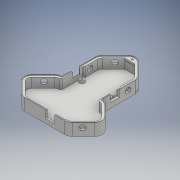
# Autodesk Inventor part: DynamicClampBottomMegaCompact
Saved by Autodesk Inventor 2017 (Build 210142000, 142)
## iProperties
Created: 2017-11-01
Part Number: DynamicClampBottomMegaCompact
Material: Generic
Document SubType Name: Modeling
Designer: andrew
Density: 1 g/cm^3
Appearance: Default
Author: andrew
Autodesk Inventor part; units mm, degrees
ref_plane "YZ Plane" through (0, 0, 0) normal (1, 0, 0) x (0, 1, 0)
ref_plane "XZ Plane" through (0, 0, 0) normal (0, 1, 0) x (-1, 0, 0)
ref_plane "XY Plane" through (0, 0, 0) normal (0, 0, 1) x (1, 0, 0)
sketch "Sketch1" plane through (0, 0, 0) normal (0, 0, 1) x (1, 0, 0)
  line L0 (64.8995, 131.8825) -> (42.1924, 154.5896)
  arc A0 (42.1924, 154.5896) -> (23.8076, 154.5896) centre (33, 145.3972) ccw
  line L1 (23.8076, 154.5896) -> (1.1005, 131.8825)
  line L2 (-3, -3) -> (69, -3) construction
  arc A1 (4.3647, 133.7325) -> (4.35, 133.7177) centre (12.85, 125.2472) ccw
  line L3 (69, 102) -> (69, 121.983)
  line L4 (-3, -3) -> (69, -3)
  arc A2 (1.1005, 131.8825) -> (-3, 121.983) centre (11, 121.983) ccw
  arc A3 (69, 121.983) -> (64.8995, 131.8825) centre (55, 121.983) ccw
  line L5 (-12.1924, 0.8076) -> (-32.3424, 20.9576)
  line L6 (-25.6012, -1.7073) -> (-34.8573, 7.5488) construction
  arc A4 (-32.3424, 39.3424) -> (-32.3424, 20.9576) centre (-23.15, 30.15) ccw
  line L7 (-32.3424, 39.3424) -> (-12.1924, 59.4924)
  arc A5 (-3, 63.3) -> (-12.1924, 59.4924) centre (-3, 50.3) ccw
  arc A6 (-12.1924, 0.8076) -> (-3, -3) centre (-3, 10) ccw
  line L8 (78.1924, 59.4924) -> (98.3424, 39.3424)
  arc A7 (98.3424, 20.9576) -> (98.3424, 39.3424) centre (89.15, 30.15) ccw
  line L9 (98.3424, 20.9576) -> (78.1924, 0.8076)
  arc A8 (69, -3) -> (78.1924, 0.8076) centre (69, 10) ccw
  arc A9 (78.1924, 59.4924) -> (69, 63.3) centre (69, 50.3) ccw
  line L10 (69, 102) -> (69, 63.3)
  line L11 (-3, 121.983) -> (-3, 63.3)
  point P0 (-37.2921, 30.15)
  point P1 (103.2921, 30.15)
  point P2 (73.1421, 60.3)
  constraints: 24 end point, 20 point on circle, 10 centre point, 3 tangent, 3 vertical, 1 collinear, 1 equal radius
extrude "Extrusion1" add sketch "Sketch1" along normal blind 3
sketch "Sketch2" plane through (0, 0, 3) normal (0, 0, 1) x (1, 0, 0)
  line L0 (65.9995, 1.253) -> (32.9995, 1.253) construction
  line L1 (32.9995, 1.253) -> (64.747, 1.253) construction
  line L2 (64.7475, 0) -> (64.7475, 1.253) construction
  line L3 (64.7475, 1.253) -> (60.9425, 1.253) construction
  line L4 (3.8431, 128.2611) -> (24.1624, 148.5804)
  line L5 (23.8076, 154.5896) -> (1.1005, 131.8825)
  line L6 (41.8376, 148.5804) -> (24.1624, 148.5804)
  line L7 (41.8376, 148.5804) -> (62.1569, 128.2611)
  line L8 (64.8995, 131.8825) -> (42.1924, 154.5896)
  arc A0 (42.1924, 154.5896) -> (23.8076, 154.5896) centre (33, 145.3972) ccw
  line L9 (-3, -3) -> (69, -3) construction
  line L10 (-3, 99) -> (0, 99) construction
  arc A1 (1.252, 128.3272) -> (1.2515, 128.3253) centre (12.85, 125.2472) ccw
  arc A2 (0.85, 125.268) -> (0.85, 125.2472) centre (12.85, 125.2472) ccw
  arc A3 (4.3647, 133.7325) -> (4.35, 133.7177) centre (12.85, 125.2472) ccw
  line L11 (1.5, 100.5) -> (1.5, 122.6043)
  line L12 (69, 102) -> (69, 121.983)
  line L13 (64.5, 122.6043) -> (64.5, 100.5)
  line L14 (64.5, 99) -> (69, 99) construction
  line L15 (-3, -3) -> (69, -3)
  line L16 (66, 99) -> (66, 99)
  arc A4 (3.8431, 128.2611) -> (1.5, 122.6043) centre (9.5, 122.6043) ccw
  arc A5 (64.5, 122.6043) -> (62.1569, 128.2611) centre (56.5, 122.6043) ccw
  arc A6 (1.1005, 131.8825) -> (-3, 121.983) centre (11, 121.983) ccw
  arc A7 (69, 121.983) -> (64.8995, 131.8825) centre (55, 121.983) ccw
  arc A8 (0.75, 99.201) -> (1.5, 100.5) centre (0, 100.5) ccw
  arc A9 (0.75, 99.201) -> (0, 97.9019) centre (1.5, 97.9019) ccw
  arc A10 (64.5, 100.5) -> (65.25, 99.201) centre (66, 100.5) ccw
  arc A11 (66, 97.9019) -> (65.25, 99.201) centre (64.5, 97.9019) ccw
  line L17 (65.9995, 1.253) -> (32.9995, 1.253) construction
  line L18 (32.9995, 1.253) -> (64.747, 1.253) construction
  line L19 (64.7475, 0) -> (64.7475, 1.253) construction
  line L20 (64.7475, 1.253) -> (60.9425, 1.253) construction
  line L21 (3.8431, 128.2611) -> (24.1624, 148.5804)
  line L22 (23.8076, 154.5896) -> (1.1005, 131.8825)
  line L23 (41.8376, 148.5804) -> (24.1624, 148.5804)
  line L24 (41.8376, 148.5804) -> (62.1569, 128.2611)
  line L25 (64.8995, 131.8825) -> (42.1924, 154.5896)
  arc A12 (42.1924, 154.5896) -> (23.8076, 154.5896) centre (33, 145.3972) ccw
  line L26 (-3, -3) -> (69, -3) construction
  line L27 (-3, 99) -> (0, 99) construction
  arc A13 (1.252, 128.3272) -> (1.2515, 128.3253) centre (12.85, 125.2472) ccw
  arc A14 (0.85, 125.268) -> (0.85, 125.2472) centre (12.85, 125.2472) ccw
  arc A15 (4.3647, 133.7325) -> (4.35, 133.7177) centre (12.85, 125.2472) ccw
  line L28 (1.5, 100.5) -> (1.5, 122.6043)
  line L29 (69, 102) -> (69, 121.983)
  line L30 (64.5, 122.6043) -> (64.5, 100.5)
  line L31 (64.5, 99) -> (69, 99) construction
  line L32 (-3, -3) -> (69, -3)
  line L33 (66, 99) -> (66, 99)
  arc A16 (3.8431, 128.2611) -> (1.5, 122.6043) centre (9.5, 122.6043) ccw
  arc A17 (64.5, 122.6043) -> (62.1569, 128.2611) centre (56.5, 122.6043) ccw
  arc A18 (1.1005, 131.8825) -> (-3, 121.983) centre (11, 121.983) ccw
  arc A19 (69, 121.983) -> (64.8995, 131.8825) centre (55, 121.983) ccw
  arc A20 (0.75, 99.201) -> (1.5, 100.5) centre (0, 100.5) ccw
  arc A21 (0.75, 99.201) -> (0, 97.9019) centre (1.5, 97.9019) ccw
  arc A22 (64.5, 100.5) -> (65.25, 99.201) centre (66, 100.5) ccw
  arc A23 (66, 97.9019) -> (65.25, 99.201) centre (64.5, 97.9019) ccw
  line L34 (-19.0039, 14.1461) -> (-22.5076, 17.6498) construction
  arc A24 (-9.0104, 3.9896) -> (-3, 1.5) centre (-3, 10) ccw
  line L35 (-34.8573, 7.5488) -> (-12.4066, 29.9994) construction
  line L36 (-9.0104, 3.9896) -> (-29.1604, 24.1396)
  line L37 (-12.1924, 0.8076) -> (-32.3424, 20.9576)
  line L38 (-25.6012, -1.7073) -> (-34.8573, 7.5488) construction
  line L39 (-23.6319, 18.7741) -> (-14.3759, 9.5181) construction
  arc A25 (-12.1924, 0.8076) -> (-3, -3) centre (-3, 10) ccw
  arc A26 (-29.1604, 36.1604) -> (-29.1604, 24.1396) centre (-23.15, 30.15) ccw
  line L40 (-26.3333, 21.3124) -> (-26.3333, 38.9876) construction
  arc A27 (-32.3424, 39.3424) -> (-32.3424, 20.9576) centre (-23.15, 30.15) ccw
  line L41 (-19.0854, 14.0646) -> (-26.3333, 21.3124) construction
  line L42 (-29.1604, 36.1604) -> (-9.0104, 56.3104)
  line L43 (-32.3424, 39.3424) -> (-12.1924, 59.4924)
  arc A28 (-3, 58.8) -> (-9.0104, 56.3104) centre (-3, 50.3) ccw
  line L44 (-8.387, 60.3) -> (4.703, 60.3) construction
  arc A29 (-3, 63.3) -> (-12.1924, 59.4924) centre (-3, 50.3) ccw
  line L45 (88.5076, 42.6502) -> (77.2823, 31.4249) construction
  line L46 (85.0039, 46.1539) -> (88.5076, 42.6502) construction
  arc A30 (75.0104, 56.3104) -> (69, 58.8) centre (69, 50.3) ccw
  line L47 (100.8573, 52.7512) -> (78.4066, 30.3006) construction
  line L48 (78.1924, 59.4924) -> (98.3424, 39.3424)
  line L49 (91.6012, 62.0073) -> (100.8573, 52.7512) construction
  arc A31 (78.1924, 59.4924) -> (69, 63.3) centre (69, 50.3) ccw
  arc A32 (95.1604, 24.1396) -> (95.1604, 36.1604) centre (89.15, 30.15) ccw
  line L50 (92.3333, 38.9876) -> (92.3333, 21.3124) construction
  arc A33 (98.3424, 20.9576) -> (98.3424, 39.3424) centre (89.15, 30.15) ccw
  line L51 (85.0854, 46.2354) -> (92.3333, 38.9876) construction
  line L52 (95.1604, 24.1396) -> (75.0104, 3.9896)
  line L53 (98.3424, 20.9576) -> (78.1924, 0.8076)
  arc A34 (69, 1.5) -> (75.0104, 3.9896) centre (69, 10) ccw
  line L54 (74.387, 0) -> (61.297, 0) construction
  arc A35 (69, -3) -> (78.1924, 0.8076) centre (69, 10) ccw
  line L55 (69, 1.5) -> (66, 0)
  line L56 (69, 58.8) -> (66, 58.8)
  line L57 (-3, 58.8) -> (0, 58.8)
  line L58 (-3, -3) -> (-3, -1.8579)
  line L59 (75.0104, 56.3104) -> (95.1604, 36.1604)
  line L60 (-3, 1.5) -> (0, 0)
  line L61 (0, 0) -> (66, 0)
  line L62 (118.9961, 116.6519) -> (118.9961, 98.6519)
  line L63 (118.9961, 116.6519) -> (136.9961, 116.6519) construction
  line L64 (0, 97.9019) -> (0, 58.8)
  line L65 (-3, 63.3) -> (-3, 121.983)
  line L66 (69, 102) -> (69, 63.3)
  line L67 (66, 97.9019) -> (66, 58.8)
  point P0 (-7.1421, 0)
  point P1 (-37.2921, 30.15)
  point P2 (73.1421, 60.3)
  point P3 (103.2921, 30.15)
  dimension "d28" = 8
  dimension "d126" = 8
  dimension "d186" = 18
  dimension "d187" = 90
  constraints: 136 end point, 76 point on circle, 36 centre point, 27 tangent, 11 point on line, 9 vertical, 8 equal radius, 5 horizontal, 3 collinear, 3 midpoint, 2 parallel, 2 perpendicular, 6 other
  measures "d28" radius of A4
  measures "d126" radius of A16
  measures "d186" distance of L62.start L62.end
  measures "d187" angle of L62 L63
extrude "Extrusion2" add sketch "Sketch2" along normal blind 17.3 contours A4 L11 A1 L4 | A0 L8 A7 L12 L66 A31 L48 A33 L53 A35 L15 A25 L37 A27 L43 A29 L65 A6 L5 picked at (9.0553, 134.1739)
sketch "Sketch3" plane through (0, 0, 20.3) normal (0, 0, 1) x (1, 0, 0)
  line L0 (66, 58.8) -> (69, 58.8) projected
  arc A0 (75.0104, 56.3104) -> (69, 58.8) centre (69, 50.3) ccw projected
  line L1 (75.0104, 56.3104) -> (95.1604, 36.1604) projected
  arc A1 (95.1604, 24.1396) -> (95.1604, 36.1604) centre (89.15, 30.15) ccw projected
  line L2 (95.1604, 24.1396) -> (75.0104, 3.9896) projected
  arc A2 (69, 1.5) -> (75.0104, 3.9896) centre (69, 10) ccw projected
  line L3 (69, 1.5) -> (66, 0) projected
  line L4 (66, 0) -> (0, 0) projected
  line L5 (0, 0) -> (-3, 1.5) projected
  arc A3 (-9.0104, 3.9896) -> (-3, 1.5) centre (-3, 10) ccw projected
  line L6 (-9.0104, 3.9896) -> (-29.1604, 24.1396) projected
  arc A4 (-29.1604, 36.1604) -> (-29.1604, 24.1396) centre (-23.15, 30.15) ccw projected
  line L7 (-29.1604, 36.1604) -> (-9.0104, 56.3104) projected
  arc A5 (-3, 58.8) -> (-9.0104, 56.3104) centre (-3, 50.3) ccw projected
  line L8 (-3, 58.8) -> (0, 58.8) projected
  arc A6 (-3, 63.3) -> (-12.1924, 59.4924) centre (-3, 50.3) ccw projected
  line L9 (-12.1924, 59.4924) -> (-32.3424, 39.3424) projected
  arc A7 (-32.3424, 39.3424) -> (-32.3424, 20.9576) centre (-23.15, 30.15) ccw projected
  line L10 (-32.3424, 20.9576) -> (-12.1924, 0.8076) projected
  arc A8 (-12.1924, 0.8076) -> (-3, -3) centre (-3, 10) ccw projected
  line L11 (-3, -3) -> (69, -3) projected
  arc A9 (69, -3) -> (78.1924, 0.8076) centre (69, 10) ccw projected
  line L12 (78.1924, 0.8076) -> (98.3424, 20.9576) projected
  arc A10 (98.3424, 20.9576) -> (98.3424, 39.3424) centre (89.15, 30.15) ccw projected
  line L13 (98.3424, 39.3424) -> (78.1924, 59.4924) projected
  arc A11 (78.1924, 59.4924) -> (69, 63.3) centre (69, 50.3) ccw projected
  line L14 (0, 58.8) -> (0, 97.9019) projected
  arc A12 (0.75, 99.201) -> (0, 97.9019) centre (1.5, 97.9019) ccw projected
  arc A13 (0.75, 99.201) -> (1.5, 100.5) centre (0, 100.5) ccw projected
  line L15 (1.5, 100.5) -> (1.5, 122.6043) projected
  arc A14 (3.8431, 128.2611) -> (1.5, 122.6043) centre (9.5, 122.6043) ccw projected
  line L16 (3.8431, 128.2611) -> (24.1624, 148.5804) projected
  line L17 (24.1624, 148.5804) -> (41.8376, 148.5804) projected
  line L18 (41.8376, 148.5804) -> (62.1569, 128.2611) projected
  arc A15 (64.5, 122.6043) -> (62.1569, 128.2611) centre (56.5, 122.6043) ccw projected
  line L19 (64.5, 122.6043) -> (64.5, 100.5) projected
  arc A16 (64.5, 100.5) -> (65.25, 99.201) centre (66, 100.5) ccw projected
  arc A17 (66, 97.9019) -> (65.25, 99.201) centre (64.5, 97.9019) ccw projected
  line L20 (66, 97.9019) -> (66, 58.8) projected
  arc A18 (42.1924, 154.5896) -> (23.8076, 154.5896) centre (33, 145.3972) ccw projected
  line L21 (23.8076, 154.5896) -> (1.1005, 131.8825) projected
  arc A19 (1.1005, 131.8825) -> (-3, 121.983) centre (11, 121.983) ccw projected
  line L22 (-3, 121.983) -> (-3, 63.3) projected
  line L23 (69, 63.3) -> (69, 121.983) projected
  arc A20 (69, 121.983) -> (64.8995, 131.8825) centre (55, 121.983) ccw projected
  line L24 (64.8995, 131.8825) -> (42.1924, 154.5896) projected
  arc A21 (-2, 62.2583) -> (-11.4853, 58.7853) centre (-3, 50.3) ccw
  line L25 (-11.4853, 58.7853) -> (-31.6353, 38.6353)
  arc A22 (-31.6353, 38.6353) -> (-31.6353, 21.6647) centre (-23.15, 30.15) ccw
  line L26 (-31.6353, 21.6647) -> (-11.4853, 1.5147)
  arc A23 (-11.4853, 1.5147) -> (-3, -2) centre (-3, 10) ccw
  line L27 (-3, -2) -> (69, -2)
  arc A24 (69, -2) -> (77.4853, 1.5147) centre (69, 10) ccw
  line L28 (77.4853, 1.5147) -> (97.6353, 21.6647)
  arc A25 (97.6353, 21.6647) -> (97.6353, 38.6353) centre (89.15, 30.15) ccw
  line L29 (97.6353, 38.6353) -> (77.4853, 58.7853)
  arc A26 (77.4853, 58.7853) -> (68, 62.2583) centre (69, 50.3) ccw
  line L30 (68, 62.2583) -> (68, 121.983)
  arc A27 (68, 121.983) -> (64.1924, 131.1754) centre (55, 121.983) ccw
  line L31 (64.1924, 131.1754) -> (41.4853, 153.8825)
  arc A28 (41.4853, 153.8825) -> (24.5147, 153.8825) centre (33, 145.3972) ccw
  line L32 (24.5147, 153.8825) -> (1.8076, 131.1754)
  arc A29 (1.8076, 131.1754) -> (-2, 121.983) centre (11, 121.983) ccw
  line L33 (-2, 121.983) -> (-2, 62.2583)
  dimension "d188" = 1
  constraints: 18 end point, 18 point on circle, 9 centre point, 17 other
  measures "d188" distance between parallel lines of L22 L33
extrude "Extrusion3" add sketch "Sketch3" along normal blind 1 contours L22 A19 L21 A18 L24 A20 L23 A11 L13 A10 L12 A9 L11 A8 L10 A7 L9 A6
sketch "Sketch4" plane through (0, 0, 3) normal (0, 0, 1) x (1, 0, 0)
  line L0 (0, 0) -> (66, 0) construction
  line L1 (66, 0) -> (66, 117) construction
  line L2 (0, 115.9019) -> (0, 0) construction
  line L3 (66, 115.9019) -> (66, 60.5) construction
  line L4 (65.9995, 1.253) -> (32.9995, 1.253) construction
  line L5 (32.9995, 1.253) -> (64.747, 1.253) construction
  line L6 (64.747, 1.253) -> (64.747, 48.238) construction
  line L7 (64.7475, 0) -> (64.7475, 1.253) construction
  line L8 (64.7475, 1.253) -> (60.9425, 1.253) construction
  line L9 (60.9425, 1.253) -> (60.9425, 5.058) construction
  line L10 (60.9425, 5.058) -> (64.7475, 5.058) construction
  line L11 (64.7475, 5.058) -> (64.7475, 1.253) construction
  circle A0 centre (60.9425, 5.058) radius 1.6
  line L12 (64.747, 95.223) -> (64.747, 48.238) construction
  line L13 (60.9425, 91.418) -> (64.7475, 91.418) construction
  circle A1 centre (60.9425, 91.418) radius 1.6
  line L14 (64.7475, 91.418) -> (64.7475, 95.223) construction
  line L15 (64.7475, 95.223) -> (60.9425, 95.223) construction
  line L16 (60.9425, 95.223) -> (60.9425, 91.418) construction
  line L17 (64.7475, 96.476) -> (64.7475, 95.223) construction
  line L18 (65.9995, 95.223) -> (32.9995, 95.223) construction
  line L19 (32.9995, 95.223) -> (64.747, 95.223) construction
  line L20 (32.9995, 95.223) -> (1.252, 95.223) construction
  line L21 (-0.0005, 95.223) -> (32.9995, 95.223) construction
  line L22 (1.2515, 91.418) -> (1.2515, 95.223) construction
  line L23 (5.0565, 91.418) -> (1.2515, 91.418) construction
  line L24 (5.0565, 95.223) -> (5.0565, 91.418) construction
  circle A2 centre (5.0565, 91.418) radius 1.6
  line L25 (1.252, 95.223) -> (1.252, 48.238) construction
  line L26 (-0.0005, 1.253) -> (32.9995, 1.253) construction
  line L27 (32.9995, 1.253) -> (1.252, 1.253) construction
  line L28 (1.252, 1.253) -> (1.252, 48.238) construction
  line L29 (5.0565, 5.058) -> (1.2515, 5.058) construction
  circle A3 centre (5.0565, 5.058) radius 1.6
  line L30 (5.0565, 1.253) -> (5.0565, 5.058) construction
  line L31 (1.2515, 5.058) -> (1.2515, 1.253) construction
  line L32 (1.2515, 1.253) -> (5.0565, 1.253) construction
  line L33 (1.2515, 0) -> (1.2515, 1.253) construction
  line L34 (1.2515, 95.223) -> (5.0565, 95.223) construction
  line L35 (1.2515, 96.476) -> (1.2515, 95.223) construction
  line L36 (32.9995, 95.223) -> (1.9995, 95.223) construction
  line L37 (1.9995, 95.223) -> (1.9995, 113.223) construction
  line L38 (1.9995, 113.223) -> (32.9995, 113.223) construction
  line L39 (32.9995, 113.223) -> (32.9995, 95.223) construction
  line L40 (63.9995, 113.223) -> (32.9995, 113.223) construction
  line L41 (63.9995, 95.223) -> (63.9995, 113.223) construction
  line L42 (3.8431, 146.2611) -> (24.1624, 166.5804)
  line L43 (23.8076, 172.5896) -> (1.1005, 149.8825)
  line L44 (41.8376, 166.5804) -> (24.1624, 166.5804)
  line L45 (41.8376, 166.5804) -> (62.1569, 146.2611)
  line L46 (64.8995, 149.8825) -> (42.1924, 172.5896)
  arc A4 (42.1924, 172.5896) -> (23.8076, 172.5896) centre (33, 163.3972) ccw
  line L47 (-3, -3) -> (69, -3) construction
  line L48 (69, -3) -> (69, 120) construction
  line L49 (-3, 117) -> (0, 117) construction
  arc A5 (1.252, 146.3272) -> (1.2515, 146.3253) centre (12.85, 143.2472) ccw
  arc A6 (0.85, 143.268) -> (0.85, 143.2472) centre (12.85, 143.2472) ccw
  arc A7 (4.3647, 151.7325) -> (4.35, 151.7177) centre (12.85, 143.2472) ccw
  line L50 (1.5, 118.5) -> (1.5, 140.6043)
  line L51 (69, 120) -> (69, 139.983)
  line L52 (64.5, 140.6043) -> (64.5, 118.5)
  line L53 (64.5, 117) -> (69, 117) construction
  line L54 (-3, -3) -> (69, -3)
  line L55 (69, 120) -> (69, -3)
  line L56 (66, 117) -> (66, 117)
  arc A8 (3.8431, 146.2611) -> (1.5, 140.6043) centre (9.5, 140.6043) ccw
  arc A9 (64.5, 140.6043) -> (62.1569, 146.2611) centre (56.5, 140.6043) ccw
  arc A10 (1.1005, 149.8825) -> (-3, 139.983) centre (11, 139.983) ccw
  arc A11 (69, 139.983) -> (64.8995, 149.8825) centre (55, 139.983) ccw
  arc A12 (0.75, 117.201) -> (1.5, 118.5) centre (0, 118.5) ccw
  arc A13 (0.75, 117.201) -> (0, 115.9019) centre (1.5, 115.9019) ccw
  line L57 (0, 115.9019) -> (0, 0)
  arc A14 (64.5, 118.5) -> (65.25, 117.201) centre (66, 118.5) ccw
  arc A15 (66, 115.9019) -> (65.25, 117.201) centre (64.5, 115.9019) ccw
  line L58 (66, 115.9019) -> (66, 0)
  line L59 (-3, -3) -> (-3, 139.983)
  circle A16 centre (5.0565, 5.058) radius 4
  circle A17 centre (60.9425, 5.058) radius 4
  circle A18 centre (5.0565, 91.418) radius 4
  circle A19 centre (60.9425, 91.418) radius 4
  dimension "d36" = 117
  dimension "d37" = 3.805
  dimension "d38" = 3.805
  dimension "d39" = 3.2
  dimension "d40" = 8
  dimension "d41" = 14
  dimension "d42" = 1.5
  dimension "d43" = 8
  dimension "d44" = 8
  dimension "d45" = 8
  dimension "d46" = 8
  constraints: 120 end point, 26 point on circle, 20 centre point, 15 tangent, 8 coincident, 6 perpendicular, 6 point on line, 5 parallel, 4 equal radius, 4 horizontal, 4 vertical, 3 collinear, 2 symmetric about line, 1 other
  measures "d36" distance of L1.end L0.end
  measures "d37" distance of L9.end L10.end
  measures "d38" distance of L8.end L9.end
  measures "d39" diameter of A0
  measures "d40" radius of A8
  measures "d41" radius of A10
  measures "d42" radius of A14
  measures "d43" diameter of A16
  measures "d44" diameter of A17
  measures "d45" diameter of A18
  measures "d46" diameter of A19
extrude "Extrusion4" add sketch "Sketch4" along normal blind 4 contours A16 | A17 | A18 | A19
sketch "Sketch6" plane through (1.1005, 131.8825, 21.3) normal (-0.7071068, 0.7071068, 0) x (0.7071068, 0.7071068, 0)
  line L0 (12.3053, 11.8312) -> (18.6412, 11.8312)
  arc A0 (12.3053, 11.8312) -> (18.6412, 11.8312) centre (15.4732, 8.0212) ccw
  line L1 (0, 21.29) -> (0, 0)
  line L2 (28.4964, 0) -> (0, 0)
  line L3 (28.4964, 21.29) -> (28.4964, 0)
  line L4 (0, 21.29) -> (28.4964, 21.29)
  point P0 (-94.0332, 21.3)
  constraints: 10 end point, 2 point on circle, 1 centre point
extrude "Extrusion6" cut sketch "Sketch6" against normal blind 10 contours L0 A0
sketch "Sketch7" plane through (42.1924, 154.5896, 21.3) normal (0.7071068, 0.7071068, 0) x (0, 0, -1)
  line L0 (11.8312, -15.9216) -> (11.8312, -22.2575)
  arc A0 (11.8312, -15.9216) -> (11.8312, -22.2575) centre (8.0212, -19.0895) ccw
  line L1 (21.29, -3.6163) -> (0, -3.6163)
  line L2 (0, -32.1127) -> (0, -3.6163)
  line L3 (21.29, -32.1127) -> (0, -32.1127)
  line L4 (21.29, -3.6163) -> (21.29, -32.1127)
  point P0 (21.3, -79.4768)
  constraints: 10 end point, 2 point on circle, 1 centre point
extrude "Extrusion7" cut sketch "Sketch7" against normal blind 10 contours L0 A0
sketch "Sketch10" plane through (0, 0, 7) normal (0, 0, 1) x (1, 0, 0)
  circle A0 centre (5.0565, 5.058) radius 1.6 projected
  circle A1 centre (5.0565, 91.418) radius 1.6 projected
  circle A2 centre (60.9425, 5.058) radius 1.6 projected
  circle A3 centre (60.9425, 91.418) radius 1.6 projected
  point P0 (0, 0)
extrude "Extrusion8" cut sketch "Sketch10" against normal blind 6
sketch "Sketch11" plane through (-3, -3, 0) normal (0, -1, 0) x (1, 0, 0)
  line L0 (4.0565, 3) -> (12.0565, 3) projected
  line L1 (6.4565, 7) -> (9.6565, 7) projected
  line L2 (12.0565, 7) -> (4.0565, 7) projected
  line L3 (62.3425, 7) -> (65.5425, 7) construction
  line L4 (67.9425, 7) -> (59.9425, 7) construction
  line L5 (4.0565, 7) -> (35.9995, 7) construction
  line L6 (4.1005, 0) -> (4.1005, 3) projected
  line L7 (35.9995, 7) -> (35.9995, 8) construction
  line L8 (35.9995, 8) -> (35.9995, 19) construction
  line L9 (53.9995, 19) -> (55.9995, 19) construction
  line L10 (55.9995, 8) -> (55.9995, 7) construction
  line L11 (35.9995, 8) -> (55.9995, 8) construction
  line L12 (35.9995, 8) -> (37.9995, 8) construction
  line L13 (37.9995, 8) -> (37.9995, 19) construction
  line L14 (55.9995, 8) -> (53.9995, 8) construction
  line L15 (53.9995, 8) -> (53.9995, 19) construction
  line L16 (37.9995, 19) -> (37.9995, 24.5991) construction
  line L17 (37.9995, 24.5991) -> (53.9995, 24.5991) construction
  line L18 (53.9995, 24.5991) -> (53.9995, 19) construction
  line L19 (37.9995, 24.5991) -> (53.9995, 24.5991)
  line L20 (53.9995, 24.5991) -> (53.9995, 8)
  line L21 (53.9995, 8) -> (37.9995, 8)
  line L22 (37.9995, 8) -> (37.9995, 24.5991)
  point P0 (3, 0)
  point P1 (4.1005, 21.3)
  point P2 (4.1005, 20.3)
  dimension "d89" = 1
  dimension "d90" = 11
  dimension "d91" = 20
  dimension "d102" = 2
  dimension "d103" = 2
  constraints: 34 end point, 9 perpendicular, 3 vertical, 2 parallel, 2 point on line, 1 horizontal
  measures "d89" distance of L5.end L7.end
  measures "d90" distance of L7.end L8.end
  measures "d91" distance of L8.end L9.end
  measures "d102" distance of L7.end L12.end
  measures "d103" distance of L10.start L14.end
extrude "Extrusion9" cut sketch "Sketch11" against normal blind 6
sketch "Sketch13" plane through (0, 0, 20.3) normal (0, 0, 1) x (1, 0, 0)
  circle A0 centre (-63.0458, -19.0499) radius 1.6
  circle A1 centre (-63.0458, -19.0499) radius 1.6
  line L0 (-71.8833, -22.7667) -> (-54.2082, -22.7667)
  line L1 (-54.2082, -22.7667) -> (-36.8854, -40.0895)
  line L2 (-34.4105, -37.6146) -> (-54.5605, -17.4646)
  arc A2 (-54.5605, -17.4646) -> (-71.5311, -17.4646) centre (-63.0458, -25.9499) ccw
  line L3 (-71.5311, -17.4646) -> (-91.6811, -37.6146)
  line L4 (-89.2062, -40.0895) -> (-71.8833, -22.7667)
  circle A3 centre (-63.0458, -19.0499) radius 1.6
  circle A4 centre (-63.0458, -19.0499) radius 1.6
  line L5 (-71.8833, -22.7667) -> (-54.2082, -22.7667)
  line L6 (-54.2082, -22.7667) -> (-36.8854, -40.0895)
  line L7 (-34.4105, -37.6146) -> (-54.5605, -17.4646)
  arc A5 (-54.5605, -17.4646) -> (-71.5311, -17.4646) centre (-63.0458, -25.9499) ccw
  line L8 (-71.5311, -17.4646) -> (-91.6811, -37.6146)
  line L9 (-89.2062, -40.0895) -> (-71.8833, -22.7667)
  circle A6 centre (33, 153.0043) radius 1.6
  line L10 (8.411, 177.13) -> (8.411, 159.13)
  point P0 (0, 0)
  dimension "d189" = 18
  constraints: 22 end point, 7 centre point, 4 point on circle, 1 vertical
  measures "d189" distance of L10.start L10.end
extrude "Extrusion11" cut sketch "Sketch13" against normal blind 12 contours A6
sketch "Sketch16" plane through (0, 0, 3) normal (0, 1, 0) x (1, 0, 0)
  line L0 (34.9995, -17.3) -> (34.9995, -5) projected
  line L1 (34.9995, -5) -> (50.9995, -5) projected
  line L2 (50.9995, -5) -> (50.9995, -17.3) projected
  line L3 (66, -17.3) -> (50.9995, -17.3) projected
  line L4 (66, 0) -> (66, -17.3) projected
  line L5 (0, 0) -> (66, 0) projected
  line L6 (0, 0) -> (0, -17.3) projected
  line L7 (34.9995, -17.3) -> (0, -17.3) projected
  line L8 (66, -17.3) -> (50.9995, -17.3) projected
  line L9 (66, -17.3) -> (0, -17.3)
  line L10 (0, -17.3) -> (0, -14.3)
  line L11 (0, -14.3) -> (66, -14.3)
  line L12 (66, -14.3) -> (66, -17.3)
  line L13 (66, 0) -> (66, -17.3) projected
  line L14 (0, -14.3) -> (66, -14.3)
  line L15 (66, -14.3) -> (66, -12.3)
  line L16 (66, -12.3) -> (0, -12.3)
  line L17 (0, -12.3) -> (0, -14.3)
  point P0 (0, 3)
  dimension "d155" = 3
  dimension "d156" = 2
  constraints: 16 end point, 4 parallel, 2 horizontal, 2 perpendicular, 2 point on line
  measures "d155" distance of L9.end L10.end
  measures "d156" distance of L15.end L14.end
extrude "Extrusion14" cut sketch "Sketch16" against normal blind 1 contours L11 L6 L16 L0 | L0 L16 L2 L11 | L2 L16 L4 L11
fillet "Fillet1" radius 3 5 edges at (66, 58.8, 11.65) (0, 58.8, 11.65) (69, 63.3, 1.5) (69, 63.3, 20.8) (69, 63.3, 11.65)
sketch "Sketch18" plane through (78.1924, 59.4924, 3) normal (0.7071068, 0.7071068, 0) x (0, 0, -1)
  arc A0 (-6.4688, -12.3053) -> (-6.4688, -18.6412) centre (-10.2788, -15.4732) ccw
  line L0 (-6.4688, -12.3053) -> (-6.4688, -18.6412)
  line L1 (3, 3.6163) -> (3, -28.4964)
  line L2 (3, 3.6163) -> (-18.3, 3.6163)
  line L3 (-18.3, -28.4964) -> (-18.3, 3.6163)
  line L4 (3, -28.4964) -> (-18.3, -28.4964)
  line L5 (3, 0) -> (3, -28.4964) projected
  line L6 (3, 0) -> (0, 0) projected
  line L7 (0, 0) -> (-18.3, 0) projected
  line L8 (3, -28.4964) -> (-18.3, -28.4964) projected
  line L9 (-14.3, 101.4294) -> (-12.3, 101.4294) projected
  line L10 (-18.3, -28.4964) -> (-18.3, 0) projected
  point P0 (3, 13.2229)
  point P1 (0, 101.4294)
  constraints: 10 end point, 2 point on circle, 1 centre point
extrude "Extrusion15" cut sketch "Sketch18" against normal blind 10 contours L0 A0
sketch "Sketch19" plane through (98.3424, 20.9576, 0) normal (0.7071068, -0.7071068, 0) x (0.7071068, 0.7071068, 0)
  line L0 (0, 0) -> (-28.4964, 0) projected
  line L1 (0, 0) -> (0, 21.3) projected
  line L2 (-28.4964, 0) -> (-28.4964, 21.3) projected
  arc A0 (-12.3053, 9.4688) -> (-18.6412, 9.4688) centre (-15.4732, 13.2788) ccw
  line L3 (-12.3053, 9.4688) -> (-18.6412, 9.4688)
  line L4 (3.6163, 0) -> (-28.4964, 0)
  line L5 (3.6163, 0) -> (3.6163, 21.3)
  line L6 (-28.4964, 21.3) -> (3.6163, 21.3)
  line L7 (-28.4964, 0) -> (-28.4964, 21.3)
  line L8 (-28.4964, 21.3) -> (0, 21.3) projected
  point P0 (-84.3578, 0)
  constraints: 10 end point, 2 point on circle, 1 centre point
extrude "Extrusion16" cut sketch "Sketch19" against normal blind 10 contours L3 A0
sketch "Sketch21" plane through (-32.3424, 39.3424, 21.3) normal (-0.7071068, 0.7071068, 0) x (0.7071068, 0.7071068, 0)
  arc A0 (12.3053, 11.8312) -> (18.6412, 11.8312) centre (15.4732, 8.0212) ccw
  line L0 (12.3053, 11.8312) -> (18.6412, 11.8312)
  line L1 (0, 21.3) -> (32.1127, 21.3)
  line L2 (0, 21.3) -> (0, 0)
  line L3 (32.1127, 0) -> (0, 0)
  line L4 (32.1127, 21.3) -> (32.1127, 0)
  point P0 (-4.9497, 21.3)
  constraints: 10 end point, 2 point on circle, 1 centre point
extrude "Extrusion17" cut sketch "Sketch21" against normal blind 10 contours L0 A0
sketch "Sketch22" plane through (-12.1924, 0.8076, 0) normal (-0.7071068, -0.7071068, 0) x (0, 0, 1)
  arc A0 (9.4688, 12.3053) -> (9.4688, 18.6412) centre (13.2788, 15.4732) ccw
  line L0 (9.4688, 12.3053) -> (9.4688, 18.6412)
  line L1 (0, 0) -> (0, 32.1127)
  line L2 (0, 0) -> (21.3, 0)
  line L3 (21.3, 32.1127) -> (21.3, 0)
  line L4 (0, 32.1127) -> (21.3, 32.1127)
  line L5 (0, 0) -> (0, 28.4964) projected
  line L6 (0, 0) -> (21.3, 0) projected
  line L7 (0, 28.4964) -> (21.3, 28.4964) projected
  line L8 (21.3, 28.4964) -> (21.3, 0) projected
  point P0 (0, -9.1924)
  constraints: 10 end point, 2 point on circle, 1 centre point
extrude "Extrusion18" cut sketch "Sketch22" against normal blind 10 contours L0 A0
chamfer "Chamfer7" distance 1 distance2 4 1 edges at (1.0565, 91.418, 3) measured on face at (0.5565, 91.418, 3)
chamfer "Chamfer8" distance 1 distance2 4 1 edges at (56.9425, 91.418, 3) measured on face at (56.4425, 91.418, 3)
chamfer "Chamfer9" distance 1 distance2 4 1 edges at (56.9425, 5.058, 3) measured on face at (56.4425, 5.058, 3)
chamfer "Chamfer10" distance 1 distance2 4 1 edges at (1.0565, 5.058, 3) measured on face at (0.5565, 5.058, 3)
sketch "Sketch26" plane through (24.1624, 148.5804, 3) normal (0, -1, 0) x (1, 0, 0)
  line L0 (7.2376, 5.3) -> (10.4376, 5.3) construction
  line L1 (17.6751, 0) -> (0, 0) construction
  line L2 (17.6751, 0) -> (17.6751, 17.3) construction
  line L3 (0, 17.3) -> (17.6751, 17.3) construction
  line L4 (0, 0) -> (0, 17.3) construction
  line L5 (10.8371, 12.3) -> (10.8371, 14.3) construction
  line L6 (-24.1624, 12.3) -> (10.8371, 12.3) construction
  line L7 (-24.1624, 14.3) -> (-24.1624, 12.3) construction
  line L8 (10.8371, 14.3) -> (-24.1624, 14.3) construction
  line L9 (18.03, 0) -> (18.03, 18.3) projected
  line L10 (0, 14.3) -> (18.03, 14.3)
  line L11 (18.03, 14.3) -> (18.03, 12.3)
  line L12 (18.03, 12.3) -> (0, 12.3)
  line L13 (0, 12.3) -> (0, 14.3)
  point P0 (-24.1624, -3)
  constraints: 8 end point, 3 point on line, 2 parallel, 1 horizontal, 1 perpendicular
extrude "Extrusion19" cut sketch "Sketch26" against normal blind 1
sketch "Sketch27" plane through (69, 121.983, 3) normal (1, 0, 0) x (0, 0, -1)
  line L0 (-23.7626, 80.661) -> (-23.7626, 62.661)
  arc A0 (-5.12, -9.4162) -> (-5.12, -15.5546) centre (-9.01, -12.4854) ccw
  line L1 (-5.12, -15.5546) -> (-5.12, -9.4162)
  line L2 (6, -25.983) -> (3, -25.983) construction
  line L3 (0, -21.483) -> (0, 0.6213)
  line L4 (0, 0.6213) -> (0, -21.483)
  line L5 (0, -21.483) -> (0, -22.782)
  line L6 (0, -22.782) -> (0, -21.483)
  line L7 (0, -22.782) -> (0, -24.081)
  line L8 (0, -24.081) -> (0, -22.782)
  line L9 (0, -24.081) -> (-17.3, -24.081)
  arc A1 (1.5, -2.3787) -> (-0.8431, 3.2782) centre (-6.5, -2.3787) ccw
  arc A2 (1.7485, 3.3423) -> (1.748, 3.3442) centre (-9.85, 0.2642) ccw
  arc A3 (2.15, 0.2642) -> (2.15, 0.285) centre (-9.85, 0.2642) ccw
  arc A4 (6, -3) -> (1.8995, 6.8995) centre (-8, -3) ccw
  line L10 (1.5, -24.483) -> (1.5, -2.3787)
  arc A5 (1.5, -24.483) -> (2.25, -25.782) centre (3, -24.483) ccw
  arc A6 (3, -27.081) -> (2.25, -25.782) centre (1.5, -27.081) ccw
  line L11 (2.99, 0) -> (-18.3, 0)
  line L12 (0, 6.2782) -> (0, 0.6213)
  line L13 (0, 0.6213) -> (0, 6.2782)
  line L14 (-0.8431, 3.2782) -> (-21.1624, 23.5975)
  line L15 (0, 6.2782) -> (0, 26.5975)
  line L16 (0, 26.5975) -> (0, 6.2782)
  line L17 (-2.0565, -47.76) -> (-2.0565, -51.565) construction
  line L18 (-2.0565, -51.565) -> (1.7485, -51.565) construction
  line L19 (1.7485, -51.565) -> (1.7485, -47.76) construction
  line L20 (-29.9995, -47.7595) -> (1.748, -47.7595) construction
  line L21 (1.748, -47.7595) -> (1.748, -94.7445) construction
  line L22 (0, -121.983) -> (0, -24.081)
  line L23 (0, -24.081) -> (0, -121.983)
  line L24 (0, -24.081) -> (0, -121.983)
  line L25 (3, -142.983) -> (-63, -142.983) construction
  line L26 (3, -27.081) -> (3, -142.983) construction
  line L27 (3, -27.081) -> (3, -142.983)
  line L28 (6, -145.983) -> (6, -3)
  line L29 (-8, -29.6705) -> (-10, -29.6705)
  line L30 (-5.5, -35.9205) -> (-5.5, -42.1705) construction
  line L31 (-10, -42.1705) -> (-8, -42.1705)
  line L32 (-25.3295, -29.6705) -> (-25.3295, -42.1705)
  line L33 (-25.3295, -42.1705) -> (-10, -42.1705)
  line L34 (-10, -29.6705) -> (-25.3295, -29.6705)
  line L35 (-17.5496, -33.081) -> (-29.5992, -33.081) construction
  line L36 (-8, -33.081) -> (-5.5, -33.081)
  line L37 (-29.9995, -47.7595) -> (1.0005, -47.7595) construction
  line L38 (3.0005, -47.7595) -> (-29.9995, -47.7595) construction
  circle A7 centre (-2.0565, -51.565) radius 1.6 construction
  line L39 (1.7485, -47.76) -> (-2.0565, -47.76) construction
  line L40 (1.7485, -46.507) -> (1.7485, -47.76) construction
  line L41 (-5.5, -42.1705) -> (-1, -42.1705) construction
  line L42 (-5.5, -42.1705) -> (-1, -42.1705)
  line L43 (-1, -35.9205) -> (-5.5, -35.9205) construction
  line L44 (-8, -64.788) -> (-8, -26.565)
  line L45 (0, -35.9205) -> (-1, -35.9205)
  line L46 (-1, -42.1705) -> (-1, -35.9205) construction
  line L47 (1.0005, -47.7595) -> (1.0005, -29.7595) construction
  line L48 (-1, -42.1705) -> (-1, -29.6705)
  line L49 (0, -29.76) -> (0, -47.7595)
  line L50 (-29.9995, -29.7595) -> (-29.9995, -47.7595) construction
  line L51 (-60.9995, -29.7595) -> (-29.9995, -29.7595) construction
  line L52 (-62.9995, -47.7595) -> (-29.9995, -47.7595) construction
  line L53 (0, -64.788) -> (-8, -64.788)
  line L54 (0, -64.788) -> (-8, -64.788) construction
  line L55 (1.748, -141.7295) -> (1.748, -94.7445) construction
  line L56 (-29.9995, -141.7295) -> (1.748, -141.7295) construction
  line L57 (3.0005, -141.7295) -> (-29.9995, -141.7295) construction
  circle A8 centre (-2.0565, -137.925) radius 1.6 construction
  line L58 (-2.0565, -141.73) -> (-2.0565, -137.925) construction
  line L59 (-2.0565, -137.925) -> (1.7485, -137.925) construction
  line L60 (6, -145.983) -> (-66, -145.983) construction
  line L61 (6, -145.983) -> (-66, -145.983)
  line L62 (1.7485, -141.73) -> (-2.0565, -141.73) construction
  line L63 (1.7485, -137.925) -> (1.7485, -141.73) construction
  line L64 (1.7485, -142.983) -> (1.7485, -141.73) construction
  line L65 (-62.9995, -141.7295) -> (-29.9995, -141.7295) construction
  line L66 (-29.9995, -141.7295) -> (-61.747, -141.7295) construction
  line L67 (-29.9995, -47.7595) -> (-61.747, -47.7595) construction
  arc A9 (-20.8076, 29.6066) -> (-39.1924, 29.6066) centre (-30, 20.4142) ccw
  line L68 (0, 36.4142) -> (-18.3, 36.4142) projected
  line L69 (0, -111.925) -> (0, -121.925) projected
  line L70 (0, -25.565) -> (0, -35.565) projected
  line L71 (0, -117.9934) -> (0, -120.483) projected
  line L72 (0, -120.483) -> (0, -121.983) projected
  line L73 (0, -121.983) -> (0, -120.483) projected
  line L74 (0, -120.483) -> (0, -117.9934) projected
  line L75 (0, -117.9934) -> (0, -97.8434) projected
  line L76 (0, -97.8434) -> (0, -85.8226) projected
  line L77 (0, -85.8226) -> (0, -65.6726) projected
  line L78 (0, -65.6726) -> (0, -63.183) projected
  line L79 (0, -60.183) -> (0, -63.183) projected
  line L80 (0, -60.183) -> (0, -24.081) projected
  line L81 (0, -24.081) -> (0, -22.782) projected
  line L82 (0, -22.782) -> (0, -21.483) projected
  line L83 (0, -21.483) -> (0, 0.6213) projected
  line L84 (0, 0.6213) -> (0, 6.2782) projected
  line L85 (0, 6.2782) -> (0, 26.5975) projected
  line L86 (0, 26.5975) -> (0, 6.2782) projected
  line L87 (0, 6.2782) -> (0, 0.6213) projected
  line L88 (0, 0.6213) -> (0, -21.483) projected
  line L89 (0, -21.483) -> (0, -22.782) projected
  line L90 (0, -22.782) -> (0, -24.081) projected
  line L91 (0, -24.081) -> (0, -60.183) projected
  line L92 (0, -63.183) -> (0, -60.183) projected
  line L93 (0, -63.183) -> (0, -65.6726) projected
  line L94 (0, -65.6726) -> (0, -85.8226) projected
  line L95 (0, -85.8226) -> (0, -97.8434) projected
  line L96 (0, -97.8434) -> (0, -117.9934) projected
  line L97 (0, -25.565) -> (0, -35.565) projected
  line L98 (0, -111.925) -> (0, -121.925) projected
  point P0 (3, -121.983)
  point P1 (0, -6.081)
  point P2 (0, -26.565)
  point P3 (3, -121.983)
  point P4 (-3.7, -102.0958)
  point P5 (0, -34.565)
  point P6 (0, -112.925)
  point P7 (0, -120.925)
  point P8 (0, -112.925)
  point P9 (0, -120.925)
  point P10 (0, -26.565)
  point P11 (0, -34.565)
  point P12 (-61.7475, -142.983)
  point P13 (-18.3, 0)
  dimension "d196" = 18
  constraints: 132 end point, 17 point on circle, 10 centre point, 6 point on line, 2 coincident, 1 vertical, 7 other
  measures "d196" distance of L0.start L0.end
extrude "Extrusion20" cut sketch "Sketch27" against normal blind 100 contours L1 A2 A0 | A2 L1 A0 | L44 L31 L33 L32 L34 L29
chamfer "Chamfer11" distance 2 angle 45 5 edges at (69, 79.8125, 20.8) (69, 79.8125, 15.65) (69, 86.0625, 11) (69, 92.3125, 15.65) (69, 92.3125, 20.8)
chamfer "Chamfer12" distance 2 angle 45 3 edges at (-3, 92.3125, 16.15) (-3, 86.0625, 11) (-3, 79.8125, 16.15)
body "Solid1"
